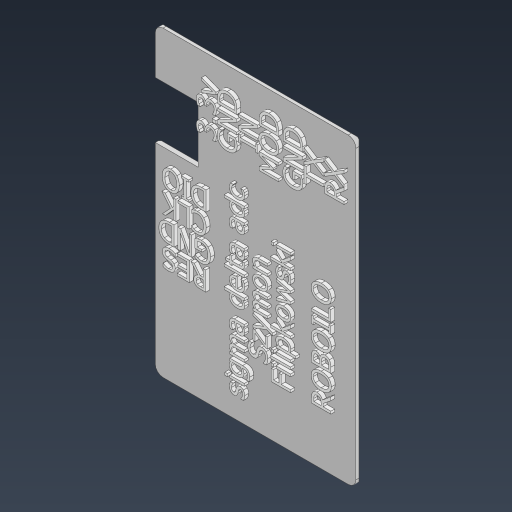
# Autodesk Inventor part: ceil
Saved by Autodesk Inventor 2023 (Build 270158000, 158)
## iProperties
Created: 2025-06-15
Part Number: ceil
Material: Generic
Document SubType Name: Modeling
Designer: szymo
Density: 1 g/cm^3
Appearance: Default
Author: szymo
Autodesk Inventor part; units mm, degrees
(part 1 of 2)
ref_plane "YZ Plane" through (0, 0, 0) normal (1, 0, 0) x (0, 1, 0)
ref_plane "XZ Plane" through (0, 0, 0) normal (0, 1, 0) x (-1, 0, 0)
ref_plane "XY Plane" through (0, 0, 0) normal (0, 0, 1) x (1, 0, 0)
sketch "Sketch1" plane through (0, 0, 0) normal (0, 0, 1) x (1, 0, 0)
  line L0 (-13.1546, 6.2718) -> (-13.1546, -19.7718) projected
  line L1 (-13.1546, -19.7718) -> (13.1639, -19.7718) projected
  line L2 (13.1639, -19.7718) -> (13.1639, 19.7718) projected
  line L3 (13.1639, 19.7718) -> (9.9954, 19.7718) projected
  line L4 (9.9954, 19.7718) -> (9.9954, 19.2718) projected
  line L5 (9.9954, 19.2718) -> (12.6639, 19.2718) projected
  line L6 (12.6639, 19.2718) -> (12.6639, -19.2718) projected
  line L7 (12.6639, -19.2718) -> (-12.6546, -19.2718) projected
  line L8 (-12.6546, -19.2718) -> (-12.6546, 6.2718) projected
  line L9 (-12.6546, 6.2718) -> (-13.1546, 6.2718) projected
  line L10 (1.8754, 19.7718) -> (-0.0446, 19.7718) projected
  line L11 (-0.0446, 19.7718) -> (-0.0446, 19.2718) projected
  line L12 (-0.0446, 19.2718) -> (1.8754, 19.2718) projected
  line L13 (1.8754, 19.2718) -> (1.8754, 19.7718) projected
  line L14 (-10.7046, 19.7718) -> (-13.1546, 19.7718) projected
  line L15 (-13.1546, 19.7718) -> (-13.1546, 13.5718) projected
  line L16 (-13.1546, 13.5718) -> (-12.6546, 13.5718) projected
  line L17 (-12.6546, 13.5718) -> (-12.6546, 19.2718) projected
  line L18 (-12.6546, 19.2718) -> (-10.7046, 19.2718) projected
  line L19 (-10.7046, 19.2718) -> (-10.7046, 19.7718) projected
  line L20 (10.1454, 19.6218) -> (13.0139, 19.6218)
  line L21 (13.0139, 19.6218) -> (13.0139, -19.6218)
  line L22 (13.0139, -19.6218) -> (-13.0046, -19.6218)
  line L23 (-13.0046, -19.6218) -> (-13.0046, 6.1218)
  line L24 (-13.0046, 6.1218) -> (-12.8046, 6.1218)
  line L25 (-12.8046, 6.1218) -> (-12.8046, -19.4218)
  line L26 (-12.8046, -19.4218) -> (12.8139, -19.4218)
  line L27 (12.8139, -19.4218) -> (12.8139, 19.4218)
  line L28 (12.8139, 19.4218) -> (10.1454, 19.4218)
  line L29 (10.1454, 19.4218) -> (10.1454, 19.6218)
  line L30 (0.1054, 19.6218) -> (1.7254, 19.6218)
  line L31 (1.7254, 19.6218) -> (1.7254, 19.4218)
  line L32 (1.7254, 19.4218) -> (0.1054, 19.4218)
  line L33 (0.1054, 19.4218) -> (0.1054, 19.6218)
  line L34 (-13.0046, 13.7218) -> (-13.0046, 19.6218)
  line L35 (-13.0046, 19.6218) -> (-10.8546, 19.6218)
  line L36 (-10.8546, 19.6218) -> (-10.8546, 19.4218)
  line L37 (-10.8546, 19.4218) -> (-12.8046, 19.4218)
  line L38 (-12.8046, 19.4218) -> (-12.8046, 13.7218)
  line L39 (-12.8046, 13.7218) -> (-13.0046, 13.7218)
  line L40 (-10.8546, 19.6218) -> (0.1054, 19.6218)
  line L41 (1.7254, 19.6218) -> (10.1454, 19.6218)
  line L42 (-13.0046, 6.1218) -> (-13.0046, 13.7218)
  line L43 (-7.9546, 13.0718) -> (-12.4546, 13.0718) projected
  line L44 (-12.4546, 13.0718) -> (-12.4546, 6.7718) projected
  line L45 (-12.4546, 6.7718) -> (-7.9546, 6.7718) projected
  line L46 (-7.9546, 6.7718) -> (-7.9546, 13.0718) projected
  line L47 (-12.9546, 6.2718) -> (-12.9546, 13.5718)
  line L48 (-12.9546, 13.5718) -> (-7.4546, 13.5718)
  line L49 (-7.4546, 13.5718) -> (-7.4546, 6.2718)
  line L50 (-7.4546, 6.2718) -> (-12.9546, 6.2718)
  point P0 (1.8754, 19.6218)
  point P1 (-0.0446, 19.6218)
  point P2 (-13.0046, 13.5718)
  point P3 (-12.6546, 6.2718)
  point P4 (-13.0046, 6.2718)
  dimension "d16" = 0.15
  dimension "d17" = 0.15
  dimension "d18" = 0.15
  dimension "d19" = 0.5
  constraints: 54 end point, 20 other
  measures "d16" distance between parallel lines of L3 L20
  measures "d17" distance between parallel lines of L10 L30
  measures "d18" distance between parallel lines of L15 L34
  measures "d19" distance between parallel lines of L44 L47
extrude "Extrusion1" add sketch "Sketch1" along normal blind 0.6 contours L9 L8 L7 L6 L5 L4 L41 L29 L28 L27 L26 L25 L24 L42 | L24 L25 L26 L27 L28 L29 L20 L21 L22 L23 | L42 L39 L38 L37 L36 L40 L19 L18 L17 L16 | L50 L49 L48 L17 L18 L19 L40 L11 L12 L13 L41 L4 L5 L6 L7 L8 | L34 L35 L36 L37 L38 L39 | L13 L12 L11 L40 L33 L32 L31 L41 | L31 L32 L33 L30
chamfer "Chamfer1" distance 0.2 angle 45 9 edges at (-5.3746, 19.6218, 0) (0.9154, 19.6218, 0) (-11.9296, 19.6218, 0) (11.5796, 19.6218, 0) (5.9354, 19.6218, 0) (-13.0046, 6.1968, 0) (-13.0046, -6.75, 0) (13.0139, 0, 0) (0.0046, -19.6218, 0)
sketch "Sketch2" plane through (0, 0, 0.6) normal (0, 0, 1) x (1, 0, 0)
  line L0 (-5.6495, -7.5123) -> (-11.7416, -7.5123) construction
  line L1 (-11.7416, -7.5123) -> (-11.7416, 5.4749) construction
  line L2 (-11.7416, 5.4749) -> (-5.6495, 5.4749) construction
  line L3 (-5.6495, 5.4749) -> (-5.6495, -7.5123) construction
  line L4 (-7.2082, 9.7459) -> (-7.2082, 17.8735) construction
  line L5 (-7.2082, 17.8735) -> (3.5331, 17.8735) construction
  line L6 (3.5331, 17.8735) -> (3.5331, 9.7459) construction
  line L7 (3.5331, 9.7459) -> (-7.2082, 9.7459) construction
  line L8 (4.1228, 9.9302) -> (4.1228, 17.763) construction
  line L9 (4.1228, 17.763) -> (11.878, 17.763) construction
  line L10 (11.878, 17.763) -> (11.878, 9.9302) construction
  line L11 (11.878, 9.9302) -> (4.1228, 9.9302) construction
  line L12 (-3.3737, -18.5812) -> (-3.3737, 9.1561) construction
  line L13 (-3.3737, 9.1561) -> (5.5235, 9.1561) construction
  line L14 (5.5235, 9.1561) -> (5.5235, -18.5812) construction
  line L15 (5.5235, -18.5812) -> (-3.3737, -18.5812) construction
  line L16 (7.7137, -12.6136) -> (7.7137, 4.051) construction
  line L17 (7.7137, 4.051) -> (10.293, 4.051) construction
  line L18 (10.293, 4.051) -> (10.293, -12.6136) construction
  line L19 (10.293, -12.6136) -> (7.7137, -12.6136) construction
  line L20 (-7.8953, -4.2727) -> (-7.4638, -4.2727)
  line L21 (-7.4638, -4.2727) -> (-6.6737, -5.2675)
  line L22 (-6.6737, -5.2675) -> (-6.2928, -5.2675)
  line L23 (-6.2928, -5.2675) -> (-6.2928, -4.2727)
  line L24 (-6.2928, -4.2727) -> (-5.9606, -4.2727)
  line L25 (-5.9606, -4.2727) -> (-5.9606, -6.7727)
  line L26 (-5.9606, -6.7727) -> (-6.6048, -6.7727)
  spline S0 degree 2 poles (-6.6048, -6.7727) (-6.8196, -6.7727) (-7.1093, -6.7261) (-7.2409, -6.6411) knots 0 0 0 1 2 2 2
  spline S1 degree 2 poles (-7.2409, -6.6411) (-7.3726, -6.556) (-7.5246, -6.2906) (-7.5246, -6.0941) knots 0 0 0 1 2 2 2
  spline S2 degree 2 poles (-7.5246, -6.0941) (-7.5246, -5.8206) (-7.245, -5.4498) (-7.0059, -5.3607) knots 0 0 0 1 2 2 2
  line L27 (-7.0059, -5.3607) -> (-7.8953, -4.2727)
  spline S3 degree 2 poles (-7.1781, -6.0677) (-7.1781, -6.1771) (-7.1012, -6.3453) (-7.0201, -6.4) knots 0 0 0 1 2 2 2
  spline S4 degree 2 poles (-7.0201, -6.4) (-6.9492, -6.4466) (-6.7608, -6.4851) (-6.623, -6.4851) knots 0 0 0 1 2 2 2
  line L28 (-6.623, -6.4851) -> (-6.2928, -6.4851)
  line L29 (-6.2928, -6.4851) -> (-6.2928, -5.545)
  line L30 (-6.2928, -5.545) -> (-6.5845, -5.545)
  spline S5 degree 2 poles (-6.5845, -5.545) (-6.7284, -5.545) (-6.9573, -5.5957) (-7.0363, -5.6747) knots 0 0 0 1 2 2 2
  spline S6 degree 2 poles (-7.0363, -5.6747) (-7.1093, -5.7436) (-7.1781, -5.9381) (-7.1781, -6.0677) knots 0 0 0 1 2 2 2
  line L31 (-8.0939, -4.2727) -> (-8.0939, -6.7727)
  line L32 (-8.0939, -6.7727) -> (-9.6579, -6.7727)
  line L33 (-9.6579, -6.7727) -> (-9.6579, -6.477)
  line L34 (-9.6579, -6.477) -> (-8.4261, -6.477)
  line L35 (-8.4261, -6.477) -> (-8.4261, -5.7922)
  line L36 (-8.4261, -5.7922) -> (-9.5748, -5.7922)
  line L37 (-9.5748, -5.7922) -> (-9.5748, -5.4964)
  line L38 (-9.5748, -5.4964) -> (-8.4261, -5.4964)
  line L39 (-8.4261, -5.4964) -> (-8.4261, -4.5685)
  line L40 (-8.4261, -4.5685) -> (-9.6579, -4.5685)
  line L41 (-9.6579, -4.5685) -> (-9.6579, -4.2727)
  line L42 (-9.6579, -4.2727) -> (-8.0939, -4.2727)
  spline S7 degree 2 poles (-10.7195, -4.2282) (-10.448, -4.2282) (-10.0671, -4.3416) (-9.899, -4.4227) knots 0 0 0 1 2 2 2
  line L43 (-9.899, -4.4227) -> (-9.899, -4.84)
  line L44 (-9.899, -4.84) -> (-9.9233, -4.84)
  spline S8 degree 2 poles (-9.9233, -4.84) (-10.0874, -4.686) (-10.5027, -4.5159) (-10.6952, -4.5159) knots 0 0 0 1 2 2 2
  spline S9 degree 2 poles (-10.6952, -4.5159) (-10.9707, -4.5159) (-11.2523, -4.7448) (-11.2523, -4.9332) knots 0 0 0 1 2 2 2
  spline S10 degree 2 poles (-11.2523, -4.9332) (-11.2523, -5.0831) (-11.1044, -5.2695) (-10.9443, -5.3161) knots 0 0 0 1 2 2 2
  spline S11 degree 2 poles (-10.9443, -5.3161) (-10.8289, -5.3485) (-10.6364, -5.3931) (-10.4926, -5.4295) knots 0 0 0 1 2 2 2
  spline S12 degree 2 poles (-10.4926, -5.4295) (-10.3629, -5.464) (-10.1583, -5.5673) (-10.0793, -5.6504) knots 0 0 0 1 2 2 2
  spline S13 degree 2 poles (-10.0793, -5.6504) (-10.0023, -5.7334) (-9.9172, -5.9563) (-9.9172, -6.1022) knots 0 0 0 1 2 2 2
  spline S14 degree 2 poles (-9.9172, -6.1022) (-9.9172, -6.406) (-10.3913, -6.8173) (-10.758, -6.8173) knots 0 0 0 1 2 2 2
  spline S15 degree 2 poles (-10.758, -6.8173) (-10.9687, -6.8173) (-11.3414, -6.7342) (-11.5015, -6.6552) knots 0 0 0 1 2 2 2
  line L45 (-11.5015, -6.6552) -> (-11.5015, -6.2582)
  line L46 (-11.5015, -6.2582) -> (-11.4772, -6.2582)
  spline S16 degree 2 poles (-11.4772, -6.2582) (-11.3576, -6.3676) (-10.9849, -6.5296) (-10.7802, -6.5296) knots 0 0 0 1 2 2 2
  spline S17 degree 2 poles (-10.7802, -6.5296) (-10.5493, -6.5296) (-10.2636, -6.3129) (-10.2636, -6.1366) knots 0 0 0 1 2 2 2
  spline S18 degree 2 poles (-10.2636, -6.1366) (-10.2636, -5.9786) (-10.4318, -5.7902) (-10.5898, -5.7476) knots 0 0 0 1 2 2 2
  spline S19 degree 2 poles (-10.5898, -5.7476) (-10.6952, -5.7193) (-11.0011, -5.6463) (-11.1024, -5.6159) knots 0 0 0 1 2 2 2
  spline S20 degree 2 poles (-11.1024, -5.6159) (-11.3597, -5.5369) (-11.5987, -5.2188) (-11.5987, -4.9859) knots 0 0 0 1 2 2 2
  spline S21 degree 2 poles (-11.5987, -4.9859) (-11.5987, -4.838) (-11.4792, -4.5543) (-11.3718, -4.4551) knots 0 0 0 1 2 2 2
  spline S22 degree 2 poles (-11.3718, -4.4551) (-11.2523, -4.3457) (-10.9484, -4.2282) (-10.7195, -4.2282) knots 0 0 0 1 2 2 2
  spline S23 degree 2 poles (-6.5349, -1.2241) (-6.2695, -1.2241) (-5.8299, -1.3862) (-5.6719, -1.5503) knots 0 0 0 1 2 2 2
  spline S24 degree 2 poles (-5.6719, -1.5503) (-5.5138, -1.7164) (-5.3457, -2.2067) (-5.3457, -2.5248) knots 0 0 0 1 2 2 2
  spline S25 degree 2 poles (-5.3457, -2.5248) (-5.3457, -2.8266) (-5.5159, -3.3047) (-5.6739, -3.4749) knots 0 0 0 1 2 2 2
  spline S26 degree 2 poles (-5.6739, -3.4749) (-5.8258, -3.639) (-6.2715, -3.8173) (-6.5369, -3.8173) knots 0 0 0 1 2 2 2
  spline S27 degree 2 poles (-6.5369, -3.8173) (-6.6646, -3.8173) (-6.8955, -3.7808) (-7.0009, -3.7484) knots 0 0 0 1 2 2 2
  spline S28 degree 2 poles (-7.0009, -3.7484) (-7.086, -3.7241) (-7.2926, -3.635) (-7.3554, -3.6026) knots 0 0 0 1 2 2 2
  line L47 (-7.3554, -3.6026) -> (-7.3554, -3.2014)
  line L48 (-7.3554, -3.2014) -> (-7.327, -3.2014)
  spline S29 degree 2 poles (-7.327, -3.2014) (-7.2642, -3.2561) (-7.1326, -3.3554) (-7.011, -3.4121) knots 0 0 0 1 2 2 2
  spline S30 degree 2 poles (-7.011, -3.4121) (-6.9097, -3.4628) (-6.6484, -3.5296) (-6.4984, -3.5296) knots 0 0 0 1 2 2 2
  spline S31 degree 2 poles (-6.4984, -3.5296) (-6.1378, -3.5296) (-5.6921, -2.9867) (-5.6921, -2.5349) knots 0 0 0 1 2 2 2
  spline S32 degree 2 poles (-5.6921, -2.5349) (-5.6921, -2.2837) (-5.8096, -1.9069) (-5.9211, -1.7772) knots 0 0 0 1 2 2 2
  spline S33 degree 2 poles (-5.9211, -1.7772) (-6.0284, -1.6475) (-6.3323, -1.5118) (-6.5228, -1.5118) knots 0 0 0 1 2 2 2
  spline S34 degree 2 poles (-6.5228, -1.5118) (-6.6625, -1.5118) (-6.9421, -1.5523) (-7.0373, -1.5928) knots 0 0 0 1 2 2 2
  line L49 (-7.0373, -1.5928) -> (-7.0373, -2.2391)
  line L50 (-7.0373, -2.2391) -> (-6.4579, -2.2391)
  line L51 (-6.4579, -2.2391) -> (-6.4579, -2.5308)
  line L52 (-6.4579, -2.5308) -> (-7.3655, -2.5308)
  line L53 (-7.3655, -2.5308) -> (-7.3655, -1.4389)
  spline S35 degree 2 poles (-7.3655, -1.4389) (-7.3027, -1.4105) (-7.088, -1.3234) (-6.9968, -1.297) knots 0 0 0 1 2 2 2
  spline S36 degree 2 poles (-6.9968, -1.297) (-6.8732, -1.2606) (-6.6747, -1.2241) (-6.5349, -1.2241) knots 0 0 0 1 2 2 2
  line L54 (-9.5718, -1.2727) -> (-9.199, -1.2727)
  line L55 (-9.199, -1.2727) -> (-8.0929, -3.4283)
  line L56 (-8.0929, -3.4283) -> (-8.0929, -1.2727)
  line L57 (-8.0929, -1.2727) -> (-7.7829, -1.2727)
  line L58 (-7.7829, -1.2727) -> (-7.7829, -3.7727)
  line L59 (-7.7829, -3.7727) -> (-8.2549, -3.7727)
  line L60 (-8.2549, -3.7727) -> (-9.2618, -1.7934)
  line L61 (-9.2618, -1.7934) -> (-9.2618, -3.7727)
  line L62 (-9.2618, -3.7727) -> (-9.5718, -3.7727)
  line L63 (-9.5718, -3.7727) -> (-9.5718, -1.2727)
  spline S37 degree 2 poles (-12.0495, -2.5207) (-12.0495, -2.1783) (-11.7719, -1.6273) (-11.539, -1.4733) knots 0 0 0 1 2 2 2
  spline S38 degree 2 poles (-11.539, -1.4733) (-11.3485, -1.3538) (-10.9575, -1.2727) (-10.6536, -1.2727) knots 0 0 0 1 2 2 2
  line L64 (-10.6536, -1.2727) -> (-10.0783, -1.2727)
  line L65 (-10.0783, -1.2727) -> (-10.0783, -3.7727)
  line L66 (-10.0783, -3.7727) -> (-10.6476, -3.7727)
  spline S39 degree 2 poles (-10.6476, -3.7727) (-11.0001, -3.7727) (-11.4012, -3.6674) (-11.543, -3.5742) knots 0 0 0 1 2 2 2
  spline S40 degree 2 poles (-11.543, -3.5742) (-11.7841, -3.4141) (-12.0495, -2.8854) (-12.0495, -2.5207) knots 0 0 0 1 2 2 2
  spline S41 degree 2 poles (-11.7031, -2.5248) (-11.7031, -2.8124) (-11.5126, -3.2197) (-11.3242, -3.3351) knots 0 0 0 1 2 2 2
  spline S42 degree 2 poles (-11.3242, -3.3351) (-11.1905, -3.4141) (-10.8886, -3.4851) (-10.6638, -3.4851) knots 0 0 0 1 2 2 2
  line L67 (-10.6638, -3.4851) -> (-10.4105, -3.4851)
  line L68 (-10.4105, -3.4851) -> (-10.4105, -1.5604)
  line L69 (-10.4105, -1.5604) -> (-10.6638, -1.5604)
  spline S43 degree 2 poles (-10.6638, -1.5604) (-10.8846, -1.5604) (-11.2189, -1.6313) (-11.3546, -1.7265) knots 0 0 0 1 2 2 2
  spline S44 degree 2 poles (-11.3546, -1.7265) (-11.5288, -1.8441) (-11.7031, -2.233) (-11.7031, -2.5248) knots 0 0 0 1 2 2 2
  spline S45 degree 2 poles (-7.0272, 1.7718) (-6.7841, 1.7718) (-6.3728, 1.6077) (-6.2229, 1.4436) knots 0 0 0 1 2 2 2
  spline S46 degree 2 poles (-6.2229, 1.4436) (-6.073, 1.2816) (-5.9089, 0.7953) (-5.9089, 0.4793) knots 0 0 0 1 2 2 2
  spline S47 degree 2 poles (-5.9089, 0.4793) (-5.9089, 0.1653) (-6.0689, -0.3007) (-6.2209, -0.4729) knots 0 0 0 1 2 2 2
  spline S48 degree 2 poles (-6.2209, -0.4729) (-6.3708, -0.6411) (-6.78, -0.8173) (-7.0333, -0.8173) knots 0 0 0 1 2 2 2
  spline S49 degree 2 poles (-7.0333, -0.8173) (-7.1589, -0.8173) (-7.3797, -0.7808) (-7.4729, -0.7525) knots 0 0 0 1 2 2 2
  spline S50 degree 2 poles (-7.4729, -0.7525) (-7.554, -0.7261) (-7.7221, -0.6512) (-7.8052, -0.6066) knots 0 0 0 1 2 2 2
  line L70 (-7.8052, -0.6066) -> (-7.8052, -0.2055)
  line L71 (-7.8052, -0.2055) -> (-7.7788, -0.2055)
  spline S51 degree 2 poles (-7.7788, -0.2055) (-7.7343, -0.246) (-7.5965, -0.3594) (-7.4972, -0.4141) knots 0 0 0 1 2 2 2
  spline S52 degree 2 poles (-7.4972, -0.4141) (-7.402, -0.4668) (-7.1771, -0.5337) (-7.0313, -0.5337) knots 0 0 0 1 2 2 2
  spline S53 degree 2 poles (-7.0313, -0.5337) (-6.8712, -0.5337) (-6.5856, -0.402) (-6.4782, -0.2764) knots 0 0 0 1 2 2 2
  spline S54 degree 2 poles (-6.4782, -0.2764) (-6.3728, -0.1488) (-6.2553, 0.2382) (-6.2553, 0.4793) knots 0 0 0 1 2 2 2
  spline S55 degree 2 poles (-6.2553, 0.4793) (-6.2553, 0.7366) (-6.3789, 1.1073) (-6.4863, 1.235) knots 0 0 0 1 2 2 2
  spline S56 degree 2 poles (-6.4863, 1.235) (-6.5916, 1.3585) (-6.8732, 1.4841) (-7.0313, 1.4841) knots 0 0 0 1 2 2 2
  spline S57 degree 2 poles (-7.0313, 1.4841) (-7.1751, 1.4841) (-7.4202, 1.4132) (-7.5155, 1.3606) knots 0 0 0 1 2 2 2
  spline S58 degree 2 poles (-7.5155, 1.3606) (-7.6066, 1.3079) (-7.7424, 1.1985) (-7.7809, 1.16) knots 0 0 0 1 2 2 2
  line L72 (-7.7809, 1.16) -> (-7.8052, 1.16)
  line L73 (-7.8052, 1.16) -> (-7.8052, 1.5571)
  spline S59 degree 2 poles (-7.8052, 1.5571) (-7.7221, 1.5956) (-7.5762, 1.6665) (-7.4729, 1.6989) knots 0 0 0 1 2 2 2
  spline S60 degree 2 poles (-7.4729, 1.6989) (-7.3635, 1.7354) (-7.1771, 1.7718) (-7.0272, 1.7718) knots 0 0 0 1 2 2 2
  line L74 (-9.5637, 1.7273) -> (-8.1151, 1.7273)
  line L75 (-8.1151, 1.7273) -> (-8.1151, -0.7727)
  line L76 (-8.1151, -0.7727) -> (-8.4474, -0.7727)
  line L77 (-8.4474, -0.7727) -> (-8.4474, 1.4315)
  line L78 (-8.4474, 1.4315) -> (-9.5637, 1.4315)
  line L79 (-9.5637, 1.4315) -> (-9.5637, 1.7273)
  line L80 (-11.6484, 1.7273) -> (-11.2168, 1.7273)
  line L81 (-11.2168, 1.7273) -> (-10.3031, 0.5644)
  line L82 (-10.3031, 0.5644) -> (-10.1573, 0.7285)
  line L83 (-10.1573, 0.7285) -> (-10.1573, 1.7273)
  line L84 (-10.1573, 1.7273) -> (-9.825, 1.7273)
  line L85 (-9.825, 1.7273) -> (-9.825, -0.7727)
  line L86 (-9.825, -0.7727) -> (-10.1573, -0.7727)
  line L87 (-10.1573, -0.7727) -> (-10.1573, 0.376)
  line L88 (-10.1573, 0.376) -> (-11.1824, -0.7727)
  line L89 (-11.1824, -0.7727) -> (-11.5876, -0.7727)
  line L90 (-11.5876, -0.7727) -> (-10.5523, 0.3435)
  line L91 (-10.5523, 0.3435) -> (-11.6484, 1.7273)
  spline S61 degree 2 poles (-7.8963, 3.4793) (-7.8963, 3.8217) (-7.6188, 4.3727) (-7.3858, 4.5267) knots 0 0 0 1 2 2 2
  spline S62 degree 2 poles (-7.3858, 4.5267) (-7.1954, 4.6462) (-6.8044, 4.7273) (-6.5005, 4.7273) knots 0 0 0 1 2 2 2
  line L92 (-6.5005, 4.7273) -> (-5.9251, 4.7273)
  line L93 (-5.9251, 4.7273) -> (-5.9251, 2.2273)
  line L94 (-5.9251, 2.2273) -> (-6.4944, 2.2273)
  spline S63 degree 2 poles (-6.4944, 2.2273) (-6.8469, 2.2273) (-7.248, 2.3326) (-7.3899, 2.4258) knots 0 0 0 1 2 2 2
  spline S64 degree 2 poles (-7.3899, 2.4258) (-7.6309, 2.5859) (-7.8963, 3.1146) (-7.8963, 3.4793) knots 0 0 0 1 2 2 2
  spline S65 degree 2 poles (-7.5499, 3.4752) (-7.5499, 3.1876) (-7.3595, 2.7803) (-7.1711, 2.6649) knots 0 0 0 1 2 2 2
  spline S66 degree 2 poles (-7.1711, 2.6649) (-7.0373, 2.5859) (-6.7355, 2.5149) (-6.5106, 2.5149) knots 0 0 0 1 2 2 2
  line L95 (-6.5106, 2.5149) -> (-6.2574, 2.5149)
  line L96 (-6.2574, 2.5149) -> (-6.2574, 4.4396)
  line L97 (-6.2574, 4.4396) -> (-6.5106, 4.4396)
  spline S67 degree 2 poles (-6.5106, 4.4396) (-6.7314, 4.4396) (-7.0657, 4.3687) (-7.2014, 4.2735) knots 0 0 0 1 2 2 2
  spline S68 degree 2 poles (-7.2014, 4.2735) (-7.3757, 4.1559) (-7.5499, 3.767) (-7.5499, 3.4752) knots 0 0 0 1 2 2 2
  line L98 (-9.1281, 4.7273) -> (-8.1597, 4.7273)
  line L99 (-8.1597, 4.7273) -> (-8.1597, 4.472)
  line L100 (-8.1597, 4.472) -> (-8.4778, 4.472)
  line L101 (-8.4778, 4.472) -> (-8.4778, 2.4825)
  line L102 (-8.4778, 2.4825) -> (-8.1597, 2.4825)
  line L103 (-8.1597, 2.4825) -> (-8.1597, 2.2273)
  line L104 (-8.1597, 2.2273) -> (-9.1281, 2.2273)
  line L105 (-9.1281, 2.2273) -> (-9.1281, 2.4825)
  line L106 (-9.1281, 2.4825) -> (-8.81, 2.4825)
  line L107 (-8.81, 2.4825) -> (-8.81, 4.472)
  line L108 (-8.81, 4.472) -> (-9.1281, 4.472)
  line L109 (-9.1281, 4.472) -> (-9.1281, 4.7273)
  spline S69 degree 2 poles (-11.308, 2.5129) (-11.4498, 2.679) (-11.6078, 3.1653) (-11.6078, 3.4773) knots 0 0 0 1 2 2 2
  spline S70 degree 2 poles (-11.6078, 3.4773) (-11.6078, 3.7812) (-11.4539, 4.2735) (-11.308, 4.4396) knots 0 0 0 1 2 2 2
  spline S71 degree 2 poles (-11.308, 4.4396) (-11.154, 4.6138) (-10.7468, 4.7799) (-10.5017, 4.7799) knots 0 0 0 1 2 2 2
  spline S72 degree 2 poles (-10.5017, 4.7799) (-10.2484, 4.7799) (-9.8433, 4.6077) (-9.6954, 4.4396) knots 0 0 0 1 2 2 2
  spline S73 degree 2 poles (-9.6954, 4.4396) (-9.5515, 4.2735) (-9.3976, 3.7852) (-9.3976, 3.4773) knots 0 0 0 1 2 2 2
  spline S74 degree 2 poles (-9.3976, 3.4773) (-9.3976, 3.1632) (-9.5535, 2.6851) (-9.6974, 2.5129) knots 0 0 0 1 2 2 2
  spline S75 degree 2 poles (-9.6974, 2.5129) (-9.8433, 2.3468) (-10.2505, 2.1746) (-10.5017, 2.1746) knots 0 0 0 1 2 2 2
  spline S76 degree 2 poles (-10.5017, 2.1746) (-10.757, 2.1746) (-11.1662, 2.3529) (-11.308, 2.5129) knots 0 0 0 1 2 2 2
  spline S77 degree 2 poles (-11.2614, 3.4773) (-11.2614, 3.2301) (-11.154, 2.8472) (-11.0568, 2.7216) knots 0 0 0 1 2 2 2
  spline S78 degree 2 poles (-11.0568, 2.7216) (-10.9575, 2.5919) (-10.6779, 2.4623) (-10.5037, 2.4623) knots 0 0 0 1 2 2 2
  spline S79 degree 2 poles (-10.5037, 2.4623) (-10.3234, 2.4623) (-10.0519, 2.5879) (-9.9486, 2.7216) knots 0 0 0 1 2 2 2
  spline S80 degree 2 poles (-9.9486, 2.7216) (-9.8493, 2.8492) (-9.744, 3.2341) (-9.744, 3.4773) knots 0 0 0 1 2 2 2
  spline S81 degree 2 poles (-9.744, 3.4773) (-9.744, 3.9696) (-10.1573, 4.4923) (-10.5037, 4.4923) knots 0 0 0 1 2 2 2
  spline S82 degree 2 poles (-10.5037, 4.4923) (-10.8501, 4.4923) (-11.2614, 3.9696) (-11.2614, 3.4773) knots 0 0 0 1 2 2 2
  spline S83 degree 2 poles (-0.9203, -15.8785) (-0.9203, -16.0669) (-1.0215, -16.393) (-1.0783, -16.5004) knots 0 0 0 1 2 2 2
  line L110 (-1.0783, -16.5004) -> (-1.4328, -16.5004)
  line L111 (-1.4328, -16.5004) -> (-1.4328, -16.4842)
  spline S84 degree 2 poles (-1.4328, -16.4842) (-1.4004, -16.4437) (-1.3234, -16.3343) (-1.2809, -16.2431) knots 0 0 0 1 2 2 2
  spline S85 degree 2 poles (-1.2809, -16.2431) (-1.2424, -16.1641) (-1.1856, -15.9696) (-1.1856, -15.8663) knots 0 0 0 1 2 2 2
  spline S86 degree 2 poles (-1.1856, -15.8663) (-1.1856, -15.7913) (-1.2201, -15.6191) (-1.2485, -15.5786) knots 0 0 0 1 2 2 2
  spline S87 degree 2 poles (-1.2485, -15.5786) (-1.2869, -15.5199) (-1.3741, -15.4672) (-1.4632, -15.4672) knots 0 0 0 1 2 2 2
  spline S88 degree 2 poles (-1.4632, -15.4672) (-1.5746, -15.4672) (-1.6901, -15.5888) (-1.7286, -15.7447) knots 0 0 0 1 2 2 2
  spline S89 degree 2 poles (-1.7286, -15.7447) (-1.7428, -15.8055) (-1.7833, -16) (-1.8056, -16.0831) knots 0 0 0 1 2 2 2
  spline S90 degree 2 poles (-1.8056, -16.0831) (-1.8684, -16.2978) (-2.1277, -16.4923) (-2.3121, -16.4923) knots 0 0 0 1 2 2 2
  spline S91 degree 2 poles (-2.3121, -16.4923) (-2.5673, -16.4923) (-2.8854, -16.1094) (-2.8854, -15.7934) knots 0 0 0 1 2 2 2
  spline S92 degree 2 poles (-2.8854, -15.7934) (-2.8854, -15.6374) (-2.8084, -15.3213) (-2.7497, -15.214) knots 0 0 0 1 2 2 2
  line L112 (-2.7497, -15.214) -> (-2.4113, -15.214)
  line L113 (-2.4113, -15.214) -> (-2.4113, -15.2302)
  spline S93 degree 2 poles (-2.4113, -15.2302) (-2.5086, -15.3517) (-2.62, -15.6475) (-2.62, -15.7994) knots 0 0 0 1 2 2 2
  spline S94 degree 2 poles (-2.62, -15.7994) (-2.62, -15.9554) (-2.4883, -16.1702) (-2.3566, -16.1702) knots 0 0 0 1 2 2 2
  spline S95 degree 2 poles (-2.3566, -16.1702) (-2.2371, -16.1702) (-2.1216, -16.0426) (-2.0852, -15.9007) knots 0 0 0 1 2 2 2
  spline S96 degree 2 poles (-2.0852, -15.9007) (-2.0669, -15.8319) (-2.0305, -15.6576) (-2.0082, -15.5624) knots 0 0 0 1 2 2 2
  spline S97 degree 2 poles (-2.0082, -15.5624) (-1.9555, -15.3558) (-1.7144, -15.1451) (-1.5057, -15.1451) knots 0 0 0 1 2 2 2
  spline S98 degree 2 poles (-1.5057, -15.1451) (-1.3842, -15.1451) (-1.1694, -15.2403) (-1.0904, -15.3335) knots 0 0 0 1 2 2 2
  spline S99 degree 2 poles (-1.0904, -15.3335) (-1.0074, -15.4328) (-0.9203, -15.686) (-0.9203, -15.8785) knots 0 0 0 1 2 2 2
  line L114 (-0.9648, -14.5292) -> (-0.9648, -14.8452)
  line L115 (-0.9648, -14.8452) -> (-2.8408, -14.8452)
  line L116 (-2.8408, -14.8452) -> (-2.8408, -14.5292)
  line L117 (-2.8408, -14.5292) -> (-0.9648, -14.5292)
  line L118 (-3.1528, -14.5069) -> (-3.1528, -14.8655)
  line L119 (-3.1528, -14.8655) -> (-3.481, -14.8655)
  line L120 (-3.481, -14.8655) -> (-3.481, -14.5069)
  line L121 (-3.481, -14.5069) -> (-3.1528, -14.5069)
  spline S100 degree 2 poles (-0.665, -13.9984) (-0.6508, -13.966) (-0.6062, -13.8424) (-0.588, -13.7634) knots 0 0 0 1 2 2 2
  spline S101 degree 2 poles (-0.588, -13.7634) (-0.5657, -13.6763) (-0.5394, -13.5284) (-0.5394, -13.4413) knots 0 0 0 1 2 2 2
  spline S102 degree 2 poles (-0.5394, -13.4413) (-0.5394, -13.2954) (-0.6164, -13.0928) (-0.6852, -13.0361) knots 0 0 0 1 2 2 2
  spline S103 degree 2 poles (-0.6852, -13.0361) (-0.7541, -12.9814) (-0.9344, -12.9388) (-1.0499, -12.9388) knots 0 0 0 1 2 2 2
  line L122 (-1.0499, -12.9388) -> (-1.214, -12.9388)
  spline S104 degree 2 poles (-1.214, -12.9388) (-1.1026, -13.0665) (-0.9972, -13.3116) (-0.9972, -13.496) knots 0 0 0 1 2 2 2
  spline S105 degree 2 poles (-0.9972, -13.496) (-0.9972, -13.8161) (-1.4733, -14.1949) (-1.9211, -14.1949) knots 0 0 0 1 2 2 2
  spline S106 degree 2 poles (-1.9211, -14.1949) (-2.154, -14.1949) (-2.5147, -14.0632) (-2.6423, -13.9538) knots 0 0 0 1 2 2 2
  spline S107 degree 2 poles (-2.6423, -13.9538) (-2.7618, -13.8485) (-2.8935, -13.5588) (-2.8935, -13.4048) knots 0 0 0 1 2 2 2
  spline S108 degree 2 poles (-2.8935, -13.4048) (-2.8935, -13.2589) (-2.8246, -13.0462) (-2.7618, -12.9388) knots 0 0 0 1 2 2 2
  line L123 (-2.7618, -12.9388) -> (-2.8408, -12.9206)
  line L124 (-2.8408, -12.9206) -> (-2.8408, -12.6228)
  line L125 (-2.8408, -12.6228) -> (-1.1796, -12.6228)
  spline S109 degree 2 poles (-1.1796, -12.6228) (-0.7015, -12.6228) (-0.2557, -13.0381) (-0.2557, -13.4656) knots 0 0 0 1 2 2 2
  spline S110 degree 2 poles (-0.2557, -13.4656) (-0.2557, -13.6033) (-0.3003, -13.891) (-0.3368, -14.0146) knots 0 0 0 1 2 2 2
  line L126 (-0.3368, -14.0146) -> (-0.665, -14.0146)
  line L127 (-0.665, -14.0146) -> (-0.665, -13.9984)
  line L128 (-1.4733, -12.9388) -> (-2.5045, -12.9388)
  spline S111 degree 2 poles (-2.5045, -12.9388) (-2.5613, -13.0563) (-2.6099, -13.2549) (-2.6099, -13.3541) knots 0 0 0 1 2 2 2
  spline S112 degree 2 poles (-2.6099, -13.3541) (-2.6099, -13.5932) (-2.2574, -13.8687) (-1.9271, -13.8687) knots 0 0 0 1 2 2 2
  spline S113 degree 2 poles (-1.9271, -13.8687) (-1.6151, -13.8687) (-1.289, -13.6601) (-1.289, -13.4251) knots 0 0 0 1 2 2 2
  spline S114 degree 2 poles (-1.289, -13.4251) (-1.289, -13.3015) (-1.3862, -13.0422) (-1.4733, -12.9388) knots 0 0 0 1 2 2 2
  line L129 (-0.9648, -10.0377) -> (-2.0507, -10.0377)
  spline S115 degree 2 poles (-2.0507, -10.0377) (-2.1804, -10.0377) (-2.4012, -10.058) (-2.462, -10.0904) knots 0 0 0 1 2 2 2
  spline S116 degree 2 poles (-2.462, -10.0904) (-2.5288, -10.1228) (-2.5937, -10.2464) (-2.5937, -10.3537) knots 0 0 0 1 2 2 2
  spline S117 degree 2 poles (-2.5937, -10.3537) (-2.5937, -10.451) (-2.4741, -10.6738) (-2.3607, -10.7913) knots 0 0 0 1 2 2 2
  spline S118 degree 2 poles (-2.3607, -10.7913) (-2.3323, -10.7893) (-2.2533, -10.7853) (-2.2006, -10.7853) knots 0 0 0 1 2 2 2
  line L130 (-2.2006, -10.7853) -> (-0.9648, -10.7853)
  line L131 (-0.9648, -10.7853) -> (-0.9648, -11.1013)
  line L132 (-0.9648, -11.1013) -> (-2.0507, -11.1013)
  spline S119 degree 2 poles (-2.0507, -11.1013) (-2.1804, -11.1013) (-2.4012, -11.1216) (-2.462, -11.154) knots 0 0 0 1 2 2 2
  spline S120 degree 2 poles (-2.462, -11.154) (-2.5288, -11.1864) (-2.5937, -11.31) (-2.5937, -11.4174) knots 0 0 0 1 2 2 2
  spline S121 degree 2 poles (-2.5937, -11.4174) (-2.5937, -11.5187) (-2.466, -11.7435) (-2.3668, -11.8489) knots 0 0 0 1 2 2 2
  line L133 (-2.3668, -11.8489) -> (-0.9648, -11.8489)
  line L134 (-0.9648, -11.8489) -> (-0.9648, -12.1649)
  line L135 (-0.9648, -12.1649) -> (-2.8408, -12.1649)
  line L136 (-2.8408, -12.1649) -> (-2.8408, -11.8489)
  line L137 (-2.8408, -11.8489) -> (-2.6342, -11.8489)
  spline S122 degree 2 poles (-2.6342, -11.8489) (-2.7578, -11.7253) (-2.8935, -11.4822) (-2.8935, -11.3363) knots 0 0 0 1 2 2 2
  spline S123 degree 2 poles (-2.8935, -11.3363) (-2.8935, -11.1702) (-2.7416, -10.9129) (-2.5694, -10.846) knots 0 0 0 1 2 2 2
  spline S124 degree 2 poles (-2.5694, -10.846) (-2.7294, -10.7022) (-2.8935, -10.4307) (-2.8935, -10.2727) knots 0 0 0 1 2 2 2
  spline S125 degree 2 poles (-2.8935, -10.2727) (-2.8935, -10.1512) (-2.8186, -9.9526) (-2.7335, -9.8797) knots 0 0 0 1 2 2 2
  spline S126 degree 2 poles (-2.7335, -9.8797) (-2.6484, -9.8047) (-2.3931, -9.7217) (-2.2006, -9.7217) knots 0 0 0 1 2 2 2
  line L138 (-2.2006, -9.7217) -> (-0.9648, -9.7217)
  line L139 (-0.9648, -9.7217) -> (-0.9648, -10.0377)
  spline S127 degree 2 poles (-1.1634, -8.2326) (-1.135, -8.2711) (-1.0337, -8.4007) (-1.0033, -8.4615) knots 0 0 0 1 2 2 2
  spline S128 degree 2 poles (-1.0033, -8.4615) (-0.9587, -8.5446) (-0.9121, -8.7006) (-0.9121, -8.8424) knots 0 0 0 1 2 2 2
  spline S129 degree 2 poles (-0.9121, -8.8424) (-0.9121, -8.9579) (-0.9993, -9.1665) (-1.0783, -9.2456) knots 0 0 0 1 2 2 2
  spline S130 degree 2 poles (-1.0783, -9.2456) (-1.1553, -9.3205) (-1.3822, -9.4117) (-1.5078, -9.4117) knots 0 0 0 1 2 2 2
  spline S131 degree 2 poles (-1.5078, -9.4117) (-1.7023, -9.4117) (-1.9778, -9.2476) (-2.0568, -9.0693) knots 0 0 0 1 2 2 2
  spline S132 degree 2 poles (-2.0568, -9.0693) (-2.1297, -8.9113) (-2.1844, -8.4818) (-2.1986, -8.2326) knots 0 0 0 1 2 2 2
  line L140 (-2.1986, -8.2326) -> (-2.2594, -8.2326)
  spline S133 degree 2 poles (-2.2594, -8.2326) (-2.3688, -8.2326) (-2.5045, -8.2994) (-2.543, -8.3602) knots 0 0 0 1 2 2 2
  spline S134 degree 2 poles (-2.543, -8.3602) (-2.5815, -8.421) (-2.6058, -8.5952) (-2.6058, -8.6884) knots 0 0 0 1 2 2 2
  spline S135 degree 2 poles (-2.6058, -8.6884) (-2.6058, -8.7978) (-2.541, -9.0936) (-2.4782, -9.2415) knots 0 0 0 1 2 2 2
  line L141 (-2.4782, -9.2415) -> (-2.4782, -9.2597)
  line L142 (-2.4782, -9.2597) -> (-2.8003, -9.2597)
  spline S136 degree 2 poles (-2.8003, -9.2597) (-2.8246, -9.1726) (-2.8854, -8.8465) (-2.8854, -8.6864) knots 0 0 0 1 2 2 2
  spline S137 degree 2 poles (-2.8854, -8.6864) (-2.8854, -8.4919) (-2.8246, -8.2265) (-2.7456, -8.1212) knots 0 0 0 1 2 2 2
  spline S138 degree 2 poles (-2.7456, -8.1212) (-2.6686, -8.0178) (-2.4235, -7.9165) (-2.2472, -7.9165) knots 0 0 0 1 2 2 2
  line L143 (-2.2472, -7.9165) -> (-0.9648, -7.9165)
  line L144 (-0.9648, -7.9165) -> (-0.9648, -8.2326)
  line L145 (-0.9648, -8.2326) -> (-1.1634, -8.2326)
  line L146 (-1.4267, -8.2326) -> (-1.9474, -8.2326)
  spline S139 degree 2 poles (-1.9474, -8.2326) (-1.9373, -8.346) (-1.9028, -8.6884) (-1.8704, -8.7958) knots 0 0 0 1 2 2 2
  spline S140 degree 2 poles (-1.8704, -8.7958) (-1.8319, -8.9214) (-1.6719, -9.0855) (-1.5301, -9.0855) knots 0 0 0 1 2 2 2
  spline S141 degree 2 poles (-1.5301, -9.0855) (-1.368, -9.0855) (-1.2039, -8.9032) (-1.2039, -8.7289) knots 0 0 0 1 2 2 2
  spline S142 degree 2 poles (-1.2039, -8.7289) (-1.2039, -8.5811) (-1.3315, -8.3379) (-1.4267, -8.2326) knots 0 0 0 1 2 2 2
  line L147 (-0.9648, -4.9567) -> (-0.9648, -5.2727)
  line L148 (-0.9648, -5.2727) -> (-1.1553, -5.2727)
  spline S143 degree 2 poles (-1.1553, -5.2727) (-1.0945, -5.3456) (-1.0134, -5.453) (-0.979, -5.5259) knots 0 0 0 1 2 2 2
  spline S144 degree 2 poles (-0.979, -5.5259) (-0.9466, -5.5928) (-0.9121, -5.7366) (-0.9121, -5.8319) knots 0 0 0 1 2 2 2
  spline S145 degree 2 poles (-0.9121, -5.8319) (-0.9121, -5.9858) (-1.0398, -6.2452) (-1.1634, -6.3363) knots 0 0 0 1 2 2 2
  spline S146 degree 2 poles (-1.1634, -6.3363) (-1.2869, -6.4275) (-1.6516, -6.5288) (-1.8886, -6.5288) knots 0 0 0 1 2 2 2
  spline S147 degree 2 poles (-1.8886, -6.5288) (-2.1358, -6.5288) (-2.4964, -6.4012) (-2.6322, -6.2897) knots 0 0 0 1 2 2 2
  spline S148 degree 2 poles (-2.6322, -6.2897) (-2.7537, -6.1864) (-2.8935, -5.8967) (-2.8935, -5.7366) knots 0 0 0 1 2 2 2
  spline S149 degree 2 poles (-2.8935, -5.7366) (-2.8935, -5.5969) (-2.8307, -5.3882) (-2.7659, -5.2727) knots 0 0 0 1 2 2 2
  line L149 (-2.7659, -5.2727) -> (-3.5762, -5.2727)
  line L150 (-3.5762, -5.2727) -> (-3.5762, -4.9567)
  line L151 (-3.5762, -4.9567) -> (-0.9648, -4.9567)
  line L152 (-1.4207, -5.2727) -> (-2.5045, -5.2727)
  spline S150 degree 2 poles (-2.5045, -5.2727) (-2.5613, -5.3902) (-2.6038, -5.5766) (-2.6038, -5.684) knots 0 0 0 1 2 2 2
  spline S151 degree 2 poles (-2.6038, -5.684) (-2.6038, -5.9271) (-2.2391, -6.2026) (-1.8947, -6.2026) knots 0 0 0 1 2 2 2
  spline S152 degree 2 poles (-1.8947, -6.2026) (-1.5625, -6.2026) (-1.212, -5.9919) (-1.212, -5.7589) knots 0 0 0 1 2 2 2
  spline S153 degree 2 poles (-1.212, -5.7589) (-1.212, -5.6353) (-1.3254, -5.3841) (-1.4207, -5.2727) knots 0 0 0 1 2 2 2
  spline S154 degree 2 poles (-0.9223, -3.6844) (-0.9223, -4.1341) (-1.4267, -4.6285) (-1.8927, -4.6285) knots 0 0 0 1 2 2 2
  spline S155 degree 2 poles (-1.8927, -4.6285) (-2.3506, -4.6285) (-2.8935, -4.1483) (-2.8935, -3.7614) knots 0 0 0 1 2 2 2
  spline S156 degree 2 poles (-2.8935, -3.7614) (-2.8935, -3.5871) (-2.7922, -3.3177) (-2.6848, -3.2184) knots 0 0 0 1 2 2 2
  spline S157 degree 2 poles (-2.6848, -3.2184) (-2.5775, -3.1171) (-2.2675, -3.0097) (-2.0426, -3.0097) knots 0 0 0 1 2 2 2
  line L153 (-2.0426, -3.0097) -> (-1.8704, -3.0097)
  line L154 (-1.8704, -3.0097) -> (-1.8704, -4.3084)
  spline S158 degree 2 poles (-1.8704, -4.3084) (-1.5442, -4.3084) (-1.1978, -3.9802) (-1.1978, -3.6884) knots 0 0 0 1 2 2 2
  spline S159 degree 2 poles (-1.1978, -3.6884) (-1.1978, -3.5851) (-1.2444, -3.3845) (-1.2809, -3.3035) knots 0 0 0 1 2 2 2
  spline S160 degree 2 poles (-1.2809, -3.3035) (-1.3214, -3.2184) (-1.3923, -3.1009) (-1.4247, -3.0624) knots 0 0 0 1 2 2 2
  line L155 (-1.4247, -3.0624) -> (-1.4247, -3.0442)
  line L156 (-1.4247, -3.0442) -> (-1.0803, -3.0442)
  spline S161 degree 2 poles (-1.0803, -3.0442) (-1.058, -3.0989) (-0.9932, -3.265) (-0.975, -3.3298) knots 0 0 0 1 2 2 2
  spline S162 degree 2 poles (-0.975, -3.3298) (-0.9486, -3.421) (-0.9223, -3.5709) (-0.9223, -3.6844) knots 0 0 0 1 2 2 2
  spline S163 degree 2 poles (-2.1115, -3.3177) (-2.2391, -3.3217) (-2.4255, -3.3744) (-2.4883, -3.4251) knots 0 0 0 1 2 2 2
  spline S164 degree 2 poles (-2.4883, -3.4251) (-2.5592, -3.4798) (-2.6342, -3.652) (-2.6342, -3.7796) knots 0 0 0 1 2 2 2
  spline S165 degree 2 poles (-2.6342, -3.7796) (-2.6342, -3.9052) (-2.5592, -4.0815) (-2.4863, -4.1544) knots 0 0 0 1 2 2 2
  spline S166 degree 2 poles (-2.4863, -4.1544) (-2.4113, -4.2253) (-2.231, -4.2982) (-2.1115, -4.3084) knots 0 0 0 1 2 2 2
  line L157 (-2.1115, -4.3084) -> (-2.1115, -3.3177)
  line L158 (-0.9648, -2.3675) -> (-0.9648, -2.6836)
  line L159 (-0.9648, -2.6836) -> (-3.5762, -2.6836)
  line L160 (-3.5762, -2.6836) -> (-3.5762, -2.3675)
  line L161 (-3.5762, -2.3675) -> (-0.9648, -2.3675)
  spline S167 degree 2 poles (-0.9284, -1.3363) (-0.9284, -1.5936) (-1.2221, -1.8833) (-1.5402, -1.8833) knots 0 0 0 1 2 2 2
  line L162 (-1.5402, -1.8833) -> (-2.5795, -1.8833)
  line L163 (-2.5795, -1.8833) -> (-2.5795, -2.096)
  line L164 (-2.5795, -2.096) -> (-2.8408, -2.096)
  line L165 (-2.8408, -2.096) -> (-2.8408, -1.8833)
  line L166 (-2.8408, -1.8833) -> (-3.3797, -1.8833)
  line L167 (-3.3797, -1.8833) -> (-3.3797, -1.5673)
  line L168 (-3.3797, -1.5673) -> (-2.8408, -1.5673)
  line L169 (-2.8408, -1.5673) -> (-2.8408, -0.9858)
  line L170 (-2.8408, -0.9858) -> (-2.5795, -0.9858)
  line L171 (-2.5795, -0.9858) -> (-2.5795, -1.5673)
  line L172 (-2.5795, -1.5673) -> (-1.6861, -1.5673)
  spline S168 degree 2 poles (-1.6861, -1.5673) (-1.5442, -1.5673) (-1.3882, -1.5571) (-1.3214, -1.5227) knots 0 0 0 1 2 2 2
  spline S169 degree 2 poles (-1.3214, -1.5227) (-1.2626, -1.4943) (-1.2039, -1.3667) (-1.2039, -1.2573) knots 0 0 0 1 2 2 2
  spline S170 degree 2 poles (-1.2039, -1.2573) (-1.2039, -1.1803) (-1.2505, -1.0365) (-1.2647, -1.0041) knots 0 0 0 1 2 2 2
  line L173 (-1.2647, -1.0041) -> (-1.2647, -0.9858)
  line L174 (-1.2647, -0.9858) -> (-0.981, -0.9858)
  spline S171 degree 2 poles (-0.981, -0.9858) (-0.9567, -1.075) (-0.9284, -1.2573) (-0.9284, -1.3363) knots 0 0 0 1 2 2 2
  spline S172 degree 2 poles (-1.1634, 0.2925) (-1.135, 0.254) (-1.0337, 0.1244) (-1.0033, 0.0636) knots 0 0 0 1 2 2 2
  spline S173 degree 2 poles (-1.0033, 0.0636) (-0.9587, -0.0195) (-0.9121, -0.1755) (-0.9121, -0.3173) knots 0 0 0 1 2 2 2
  spline S174 degree 2 poles (-0.9121, -0.3173) (-0.9121, -0.4328) (-0.9993, -0.6414) (-1.0783, -0.7204) knots 0 0 0 1 2 2 2
  spline S175 degree 2 poles (-1.0783, -0.7204) (-1.1553, -0.7954) (-1.3822, -0.8866) (-1.5078, -0.8866) knots 0 0 0 1 2 2 2
  spline S176 degree 2 poles (-1.5078, -0.8866) (-1.7023, -0.8866) (-1.9778, -0.7225) (-2.0568, -0.5442) knots 0 0 0 1 2 2 2
  spline S177 degree 2 poles (-2.0568, -0.5442) (-2.1297, -0.3862) (-2.1844, 0.0433) (-2.1986, 0.2925) knots 0 0 0 1 2 2 2
  line L175 (-2.1986, 0.2925) -> (-2.2594, 0.2925)
  spline S178 degree 2 poles (-2.2594, 0.2925) (-2.3688, 0.2925) (-2.5045, 0.2257) (-2.543, 0.1649) knots 0 0 0 1 2 2 2
  spline S179 degree 2 poles (-2.543, 0.1649) (-2.5815, 0.1041) (-2.6058, -0.0701) (-2.6058, -0.1633) knots 0 0 0 1 2 2 2
  spline S180 degree 2 poles (-2.6058, -0.1633) (-2.6058, -0.2727) (-2.541, -0.5685) (-2.4782, -0.7164) knots 0 0 0 1 2 2 2
  line L176 (-2.4782, -0.7164) -> (-2.4782, -0.7346)
  line L177 (-2.4782, -0.7346) -> (-2.8003, -0.7346)
  spline S181 degree 2 poles (-2.8003, -0.7346) (-2.8246, -0.6475) (-2.8854, -0.3213) (-2.8854, -0.1613) knots 0 0 0 1 2 2 2
  spline S182 degree 2 poles (-2.8854, -0.1613) (-2.8854, 0.0332) (-2.8246, 0.2986) (-2.7456, 0.404) knots 0 0 0 1 2 2 2
  spline S183 degree 2 poles (-2.7456, 0.404) (-2.6686, 0.5073) (-2.4235, 0.6086) (-2.2472, 0.6086) knots 0 0 0 1 2 2 2
  line L178 (-2.2472, 0.6086) -> (-0.9648, 0.6086)
  line L179 (-0.9648, 0.6086) -> (-0.9648, 0.2925)
  line L180 (-0.9648, 0.2925) -> (-1.1634, 0.2925)
  line L181 (-1.4267, 0.2925) -> (-1.9474, 0.2925)
  spline S184 degree 2 poles (-1.9474, 0.2925) (-1.9373, 0.1791) (-1.9028, -0.1633) (-1.8704, -0.2707) knots 0 0 0 1 2 2 2
  spline S185 degree 2 poles (-1.8704, -0.2707) (-1.8319, -0.3963) (-1.6719, -0.5604) (-1.5301, -0.5604) knots 0 0 0 1 2 2 2
  spline S186 degree 2 poles (-1.5301, -0.5604) (-1.368, -0.5604) (-1.2039, -0.3781) (-1.2039, -0.2038) knots 0 0 0 1 2 2 2
  spline S187 degree 2 poles (-1.2039, -0.2038) (-1.2039, -0.0559) (-1.3315, 0.1872) (-1.4267, 0.2925) knots 0 0 0 1 2 2 2
  spline S188 degree 2 poles (-1.1634, 3.1714) (-1.135, 3.1329) (-1.0337, 3.0032) (-1.0033, 2.9424) knots 0 0 0 1 2 2 2
  spline S189 degree 2 poles (-1.0033, 2.9424) (-0.9587, 2.8594) (-0.9121, 2.7034) (-0.9121, 2.5616) knots 0 0 0 1 2 2 2
  spline S190 degree 2 poles (-0.9121, 2.5616) (-0.9121, 2.4461) (-0.9993, 2.2374) (-1.0783, 2.1584) knots 0 0 0 1 2 2 2
  spline S191 degree 2 poles (-1.0783, 2.1584) (-1.1553, 2.0835) (-1.3822, 1.9923) (-1.5078, 1.9923) knots 0 0 0 1 2 2 2
  spline S192 degree 2 poles (-1.5078, 1.9923) (-1.7023, 1.9923) (-1.9778, 2.1564) (-2.0568, 2.3347) knots 0 0 0 1 2 2 2
  spline S193 degree 2 poles (-2.0568, 2.3347) (-2.1297, 2.4927) (-2.1844, 2.9222) (-2.1986, 3.1714) knots 0 0 0 1 2 2 2
  line L182 (-2.1986, 3.1714) -> (-2.2594, 3.1714)
  spline S194 degree 2 poles (-2.2594, 3.1714) (-2.3688, 3.1714) (-2.5045, 3.1045) (-2.543, 3.0437) knots 0 0 0 1 2 2 2
  spline S195 degree 2 poles (-2.543, 3.0437) (-2.5815, 2.983) (-2.6058, 2.8087) (-2.6058, 2.7155) knots 0 0 0 1 2 2 2
  spline S196 degree 2 poles (-2.6058, 2.7155) (-2.6058, 2.6061) (-2.541, 2.3104) (-2.4782, 2.1625) knots 0 0 0 1 2 2 2
  line L183 (-2.4782, 2.1625) -> (-2.4782, 2.1442)
  line L184 (-2.4782, 2.1442) -> (-2.8003, 2.1442)
  spline S197 degree 2 poles (-2.8003, 2.1442) (-2.8246, 2.2313) (-2.8854, 2.5575) (-2.8854, 2.7176) knots 0 0 0 1 2 2 2
  spline S198 degree 2 poles (-2.8854, 2.7176) (-2.8854, 2.9121) (-2.8246, 3.1775) (-2.7456, 3.2828) knots 0 0 0 1 2 2 2
  spline S199 degree 2 poles (-2.7456, 3.2828) (-2.6686, 3.3861) (-2.4235, 3.4874) (-2.2472, 3.4874) knots 0 0 0 1 2 2 2
  line L185 (-2.2472, 3.4874) -> (-0.9648, 3.4874)
  line L186 (-0.9648, 3.4874) -> (-0.9648, 3.1714)
  line L187 (-0.9648, 3.1714) -> (-1.1634, 3.1714)
  line L188 (-1.4267, 3.1714) -> (-1.9474, 3.1714)
  spline S200 degree 2 poles (-1.9474, 3.1714) (-1.9373, 3.0579) (-1.9028, 2.7155) (-1.8704, 2.6082) knots 0 0 0 1 2 2 2
  spline S201 degree 2 poles (-1.8704, 2.6082) (-1.8319, 2.4826) (-1.6719, 2.3185) (-1.5301, 2.3185) knots 0 0 0 1 2 2 2
  spline S202 degree 2 poles (-1.5301, 2.3185) (-1.368, 2.3185) (-1.2039, 2.5008) (-1.2039, 2.675) knots 0 0 0 1 2 2 2
  spline S203 degree 2 poles (-1.2039, 2.675) (-1.2039, 2.8229) (-1.3315, 3.066) (-1.4267, 3.1714) knots 0 0 0 1 2 2 2
  line L189 (-0.9648, 5.3736) -> (-0.9648, 5.0575)
  line L190 (-0.9648, 5.0575) -> (-1.1553, 5.0575)
  spline S204 degree 2 poles (-1.1553, 5.0575) (-1.0945, 4.9846) (-1.0134, 4.8772) (-0.979, 4.8043) knots 0 0 0 1 2 2 2
  spline S205 degree 2 poles (-0.979, 4.8043) (-0.9466, 4.7374) (-0.9121, 4.5936) (-0.9121, 4.4984) knots 0 0 0 1 2 2 2
  spline S206 degree 2 poles (-0.9121, 4.4984) (-0.9121, 4.3444) (-1.0398, 4.0851) (-1.1634, 3.9939) knots 0 0 0 1 2 2 2
  spline S207 degree 2 poles (-1.1634, 3.9939) (-1.2869, 3.9027) (-1.6516, 3.8014) (-1.8886, 3.8014) knots 0 0 0 1 2 2 2
  spline S208 degree 2 poles (-1.8886, 3.8014) (-2.1358, 3.8014) (-2.4964, 3.9291) (-2.6322, 4.0405) knots 0 0 0 1 2 2 2
  spline S209 degree 2 poles (-2.6322, 4.0405) (-2.7537, 4.1438) (-2.8935, 4.4335) (-2.8935, 4.5936) knots 0 0 0 1 2 2 2
  spline S210 degree 2 poles (-2.8935, 4.5936) (-2.8935, 4.7334) (-2.8307, 4.942) (-2.7659, 5.0575) knots 0 0 0 1 2 2 2
  line L191 (-2.7659, 5.0575) -> (-3.5762, 5.0575)
  line L192 (-3.5762, 5.0575) -> (-3.5762, 5.3736)
  line L193 (-3.5762, 5.3736) -> (-0.9648, 5.3736)
  line L194 (-1.4207, 5.0575) -> (-2.5045, 5.0575)
  spline S211 degree 2 poles (-2.5045, 5.0575) (-2.5613, 4.94) (-2.6038, 4.7536) (-2.6038, 4.6463) knots 0 0 0 1 2 2 2
  spline S212 degree 2 poles (-2.6038, 4.6463) (-2.6038, 4.4031) (-2.2391, 4.1276) (-1.8947, 4.1276) knots 0 0 0 1 2 2 2
  spline S213 degree 2 poles (-1.8947, 4.1276) (-1.5625, 4.1276) (-1.212, 4.3383) (-1.212, 4.5713) knots 0 0 0 1 2 2 2
  spline S214 degree 2 poles (-1.212, 4.5713) (-1.212, 4.6949) (-1.3254, 4.9461) (-1.4207, 5.0575) knots 0 0 0 1 2 2 2
  spline S215 degree 2 poles (-0.9223, 6.577) (-0.9223, 6.3825) (-1.0418, 6.0604) (-1.1634, 5.9449) knots 0 0 0 1 2 2 2
  spline S216 degree 2 poles (-1.1634, 5.9449) (-1.2829, 5.8294) (-1.6516, 5.7018) (-1.8988, 5.7018) knots 0 0 0 1 2 2 2
  spline S217 degree 2 poles (-1.8988, 5.7018) (-2.1459, 5.7018) (-2.5066, 5.8335) (-2.6281, 5.9449) knots 0 0 0 1 2 2 2
  spline S218 degree 2 poles (-2.6281, 5.9449) (-2.7517, 6.0563) (-2.8834, 6.3865) (-2.8834, 6.577) knots 0 0 0 1 2 2 2
  spline S219 degree 2 poles (-2.8834, 6.577) (-2.8834, 6.7309) (-2.7963, 7.0186) (-2.7395, 7.13) knots 0 0 0 1 2 2 2
  line L195 (-2.7395, 7.13) -> (-2.385, 7.13)
  line L196 (-2.385, 7.13) -> (-2.385, 7.1118)
  spline S220 degree 2 poles (-2.385, 7.1118) (-2.4134, 7.0774) (-2.4863, 6.972) (-2.5248, 6.8971) knots 0 0 0 1 2 2 2
  spline S221 degree 2 poles (-2.5248, 6.8971) (-2.5572, 6.8302) (-2.6079, 6.6519) (-2.6079, 6.5709) knots 0 0 0 1 2 2 2
  spline S222 degree 2 poles (-2.6079, 6.5709) (-2.6079, 6.3258) (-2.2371, 6.0279) (-1.8988, 6.0279) knots 0 0 0 1 2 2 2
  spline S223 degree 2 poles (-1.8988, 6.0279) (-1.5686, 6.0279) (-1.1978, 6.3156) (-1.1978, 6.5709) knots 0 0 0 1 2 2 2
  spline S224 degree 2 poles (-1.1978, 6.5709) (-1.1978, 6.7249) (-1.3254, 7.0044) (-1.4247, 7.1118) knots 0 0 0 1 2 2 2
  line L197 (-1.4247, 7.1118) -> (-1.4247, 7.13)
  line L198 (-1.4247, 7.13) -> (-1.0702, 7.13)
  spline S225 degree 2 poles (-1.0702, 7.13) (-1.0479, 7.0835) (-0.9851, 6.9416) (-0.9709, 6.8849) knots 0 0 0 1 2 2 2
  spline S226 degree 2 poles (-0.9709, 6.8849) (-0.9466, 6.8039) (-0.9223, 6.6762) (-0.9223, 6.577) knots 0 0 0 1 2 2 2
  spline S227 degree 2 poles (2.0797, -10.2109) (2.0797, -10.4824) (1.9663, -10.8633) (1.8853, -11.0314) knots 0 0 0 1 2 2 2
  line L199 (1.8853, -11.0314) -> (1.4679, -11.0314)
  line L200 (1.4679, -11.0314) -> (1.4679, -11.0071)
  spline S228 degree 2 poles (1.4679, -11.0071) (1.6219, -10.843) (1.7921, -10.4277) (1.7921, -10.2352) knots 0 0 0 1 2 2 2
  spline S229 degree 2 poles (1.7921, -10.2352) (1.7921, -9.9597) (1.5631, -9.6781) (1.3747, -9.6781) knots 0 0 0 1 2 2 2
  spline S230 degree 2 poles (1.3747, -9.6781) (1.2248, -9.6781) (1.0384, -9.826) (0.9918, -9.986) knots 0 0 0 1 2 2 2
  spline S231 degree 2 poles (0.9918, -9.986) (0.9594, -10.1015) (0.9148, -10.294) (0.8784, -10.4378) knots 0 0 0 1 2 2 2
  spline S232 degree 2 poles (0.8784, -10.4378) (0.8439, -10.5675) (0.7406, -10.7721) (0.6575, -10.8511) knots 0 0 0 1 2 2 2
  spline S233 degree 2 poles (0.6575, -10.8511) (0.5745, -10.9281) (0.3516, -11.0132) (0.2058, -11.0132) knots 0 0 0 1 2 2 2
  spline S234 degree 2 poles (0.2058, -11.0132) (-0.0981, -11.0132) (-0.5094, -10.5391) (-0.5094, -10.1724) knots 0 0 0 1 2 2 2
  spline S235 degree 2 poles (-0.5094, -10.1724) (-0.5094, -9.9617) (-0.4263, -9.589) (-0.3473, -9.4289) knots 0 0 0 1 2 2 2
  line L201 (-0.3473, -9.4289) -> (0.0498, -9.4289)
  line L202 (0.0498, -9.4289) -> (0.0498, -9.4532)
  spline S236 degree 2 poles (0.0498, -9.4532) (-0.0596, -9.5727) (-0.2217, -9.9455) (-0.2217, -10.1501) knots 0 0 0 1 2 2 2
  spline S237 degree 2 poles (-0.2217, -10.1501) (-0.2217, -10.3811) (-0.0049, -10.6668) (0.1713, -10.6668) knots 0 0 0 1 2 2 2
  spline S238 degree 2 poles (0.1713, -10.6668) (0.3293, -10.6668) (0.5178, -10.4986) (0.5603, -10.3406) knots 0 0 0 1 2 2 2
  spline S239 degree 2 poles (0.5603, -10.3406) (0.5887, -10.2352) (0.6616, -9.9293) (0.692, -9.828) knots 0 0 0 1 2 2 2
  spline S240 degree 2 poles (0.692, -9.828) (0.771, -9.5707) (1.0891, -9.3317) (1.322, -9.3317) knots 0 0 0 1 2 2 2
  spline S241 degree 2 poles (1.322, -9.3317) (1.4699, -9.3317) (1.7536, -9.4512) (1.8528, -9.5586) knots 0 0 0 1 2 2 2
  spline S242 degree 2 poles (1.8528, -9.5586) (1.9622, -9.6781) (2.0797, -9.982) (2.0797, -10.2109) knots 0 0 0 1 2 2 2
  line L203 (2.0352, -7.7859) -> (2.0352, -9.1635)
  line L204 (2.0352, -9.1635) -> (1.8002, -9.1635)
  line L205 (1.8002, -9.1635) -> (0.4185, -8.183)
  line L206 (0.4185, -8.183) -> (0.4185, -9.123)
  line L207 (0.4185, -9.123) -> (0.1592, -9.123)
  line L208 (0.1592, -9.123) -> (0.1592, -7.8041)
  line L209 (0.1592, -7.8041) -> (0.384, -7.8041)
  line L210 (0.384, -7.8041) -> (1.7698, -8.7887)
  line L211 (1.7698, -8.7887) -> (1.7698, -7.7859)
  line L212 (1.7698, -7.7859) -> (2.0352, -7.7859)
  line L213 (0.1592, -6.0172) -> (2.726, -7.0262)
  line L214 (2.726, -7.0262) -> (2.726, -7.3645)
  line L215 (2.726, -7.3645) -> (1.944, -7.0282)
  line L216 (1.944, -7.0282) -> (0.1592, -7.7089)
  line L217 (0.1592, -7.7089) -> (0.1592, -7.3685)
  line L218 (0.1592, -7.3685) -> (1.549, -6.856)
  line L219 (1.549, -6.856) -> (0.1592, -6.3454)
  line L220 (0.1592, -6.3454) -> (0.1592, -6.0172)
  line L221 (2.0352, -3.6509) -> (0.9493, -3.6509)
  spline S243 degree 2 poles (0.9493, -3.6509) (0.8196, -3.6509) (0.5988, -3.6712) (0.538, -3.7036) knots 0 0 0 1 2 2 2
  spline S244 degree 2 poles (0.538, -3.7036) (0.4712, -3.736) (0.4063, -3.8596) (0.4063, -3.967) knots 0 0 0 1 2 2 2
  spline S245 degree 2 poles (0.4063, -3.967) (0.4063, -4.0642) (0.5259, -4.2871) (0.6393, -4.4046) knots 0 0 0 1 2 2 2
  spline S246 degree 2 poles (0.6393, -4.4046) (0.6677, -4.4026) (0.7467, -4.3985) (0.7994, -4.3985) knots 0 0 0 1 2 2 2
  line L222 (0.7994, -4.3985) -> (2.0352, -4.3985)
  line L223 (2.0352, -4.3985) -> (2.0352, -4.7146)
  line L224 (2.0352, -4.7146) -> (0.9493, -4.7146)
  spline S247 degree 2 poles (0.9493, -4.7146) (0.8196, -4.7146) (0.5988, -4.7348) (0.538, -4.7672) knots 0 0 0 1 2 2 2
  spline S248 degree 2 poles (0.538, -4.7672) (0.4712, -4.7997) (0.4063, -4.9232) (0.4063, -5.0306) knots 0 0 0 1 2 2 2
  spline S249 degree 2 poles (0.4063, -5.0306) (0.4063, -5.1319) (0.534, -5.3568) (0.6332, -5.4621) knots 0 0 0 1 2 2 2
  line L225 (0.6332, -5.4621) -> (2.0352, -5.4621)
  line L226 (2.0352, -5.4621) -> (2.0352, -5.7782)
  line L227 (2.0352, -5.7782) -> (0.1592, -5.7782)
  line L228 (0.1592, -5.7782) -> (0.1592, -5.4621)
  line L229 (0.1592, -5.4621) -> (0.3658, -5.4621)
  spline S250 degree 2 poles (0.3658, -5.4621) (0.2422, -5.3386) (0.1065, -5.0954) (0.1065, -4.9496) knots 0 0 0 1 2 2 2
  spline S251 degree 2 poles (0.1065, -4.9496) (0.1065, -4.7834) (0.2584, -4.5262) (0.4306, -4.4593) knots 0 0 0 1 2 2 2
  spline S252 degree 2 poles (0.4306, -4.4593) (0.2706, -4.3155) (0.1065, -4.044) (0.1065, -3.886) knots 0 0 0 1 2 2 2
  spline S253 degree 2 poles (0.1065, -3.886) (0.1065, -3.7644) (0.1814, -3.5659) (0.2665, -3.4929) knots 0 0 0 1 2 2 2
  spline S254 degree 2 poles (0.2665, -3.4929) (0.3516, -3.418) (0.6069, -3.3349) (0.7994, -3.3349) knots 0 0 0 1 2 2 2
  line L230 (0.7994, -3.3349) -> (2.0352, -3.3349)
  line L231 (2.0352, -3.3349) -> (2.0352, -3.6509)
  spline S255 degree 2 poles (1.0972, -1.3495) (1.5712, -1.3495) (2.0879, -1.8053) (2.0879, -2.1862) knots 0 0 0 1 2 2 2
  spline S256 degree 2 poles (2.0879, -2.1862) (2.0879, -2.5772) (1.555, -3.0249) (1.0972, -3.0249) knots 0 0 0 1 2 2 2
  spline S257 degree 2 poles (1.0972, -3.0249) (0.6272, -3.0249) (0.1065, -2.563) (0.1065, -2.1862) knots 0 0 0 1 2 2 2
  spline S258 degree 2 poles (0.1065, -2.1862) (0.1065, -1.8053) (0.6251, -1.3495) (1.0972, -1.3495) knots 0 0 0 1 2 2 2
  spline S259 degree 2 poles (1.0972, -1.6757) (0.7325, -1.6757) (0.378, -1.9411) (0.378, -2.1862) knots 0 0 0 1 2 2 2
  spline S260 degree 2 poles (0.378, -2.1862) (0.378, -2.4313) (0.7325, -2.6988) (1.0972, -2.6988) knots 0 0 0 1 2 2 2
  spline S261 degree 2 poles (1.0972, -2.6988) (1.4517, -2.6988) (1.8164, -2.4313) (1.8164, -2.1862) knots 0 0 0 1 2 2 2
  spline S262 degree 2 poles (1.8164, -2.1862) (1.8164, -1.9431) (1.4578, -1.6757) (1.0972, -1.6757) knots 0 0 0 1 2 2 2
  line L232 (2.0352, 0.4475) -> (2.0352, 0.1315)
  line L233 (2.0352, 0.1315) -> (0.9655, 0.1315)
  spline S263 degree 2 poles (0.9655, 0.1315) (0.8358, 0.1315) (0.613, 0.1072) (0.5461, 0.0707) knots 0 0 0 1 2 2 2
  spline S264 degree 2 poles (0.5461, 0.0707) (0.4752, 0.0322) (0.4063, -0.1056) (0.4063, -0.2231) knots 0 0 0 1 2 2 2
  spline S265 degree 2 poles (0.4063, -0.2231) (0.4063, -0.3406) (0.5319, -0.5898) (0.6332, -0.7093) knots 0 0 0 1 2 2 2
  line L234 (0.6332, -0.7093) -> (2.0352, -0.7093)
  line L235 (2.0352, -0.7093) -> (2.0352, -1.0253)
  line L236 (2.0352, -1.0253) -> (0.1592, -1.0253)
  line L237 (0.1592, -1.0253) -> (0.1592, -0.7093)
  line L238 (0.1592, -0.7093) -> (0.3678, -0.7093)